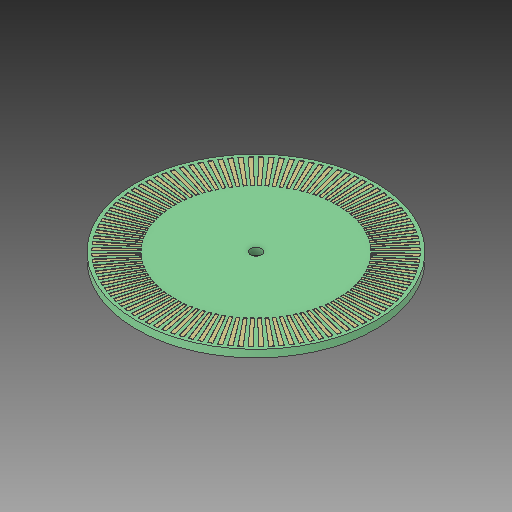
# Autodesk Inventor part: Encoder Wheel (G16)
Saved by Autodesk Inventor 2018 (Build 220112000, 112)
## iProperties
Created: 2018-01-25
Part Number: Encoder Wheel (G16)
Material: PPS Plastic
Document SubType Name: Modeling
Designer: Moochster
Density: 1.637 g/cm^3
Appearance: Smooth - White
Mass: 4.28771 g
Surface Area: 41.535 cm^2
Volume: 2.61925 cm^3
Author: Moochster
Autodesk Inventor part; units mm, degrees
ref_plane "YZ Plane" through (0, 0, 0) normal (1, 0, 0) x (0, 1, 0)
ref_plane "XZ Plane" through (0, 0, 0) normal (0, 1, 0) x (-1, 0, 0)
ref_plane "XY Plane" through (0, 0, 0) normal (0, 0, 1) x (1, 0, 0)
sketch "Sketch1" plane through (0, 0, 0) normal (0, 1, 0) x (-1, 0, 0)
  circle A0 centre (0, 0) radius 24
  circle A1 centre (0, 0) radius 1.115
  dimension "d0" = 48
  dimension "d1" = 2.23
  constraints: 2 centre point, 2 coincident
  measures "d0" diameter of A0
  measures "d1" diameter of A1
extrude "Extrusion1" add sketch "Sketch1" along normal blind 1.5
sketch "Sketch2" plane through (0, 1.5, 0) normal (0, 1, 0) x (1, 0, 0)
  circle A0 centre (0, 0) radius 24 projected
  circle A1 centre (0, 0) radius 23.3
  circle A2 centre (0, 0) radius 16.3
  line L0 (0.2623, 16.2979) -> (0.375, 23.297)
  line L1 (-0.375, 23.297) -> (-0.2623, 16.2979)
  dimension "d4" = 0.7
  dimension "d5" = 7
  dimension "d6" = 0.75
  dimension "d12" = 0.5247
  constraints: 4 end point, 4 point on circle, 2 centre point, 2 horizontal alignment, 1 point on line
  measures "d4" radial gap between concentric circles of A0 A1
  measures "d5" radial gap between concentric circles of A1 A2
  measures "d6" distance of L1.start L0.end
  measures "d12" distance of L0.start L1.end
extrude "Extrusion2" cut sketch "Sketch2" against normal blind 0.1 contours L0 A2 L1 A1 picked at (0.2541, 20.9648)
pattern_circular "Circular Pattern1" count 100 over 360 about axis through (0, 0, 0) along (0, 1, 0) of "Extrusion2"
ref_plane "Work Plane1" through (0, 0.75, 0) normal (0, 1, 0) x (1, 0, 0)
mirror "Mirror1" about plane through (0, 0.75, 0) normal (0, 1, 0) of "Extrusion2", "Circular Pattern1"
body "Solid1"
